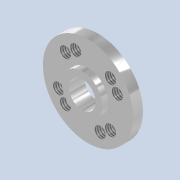
# Autodesk Inventor part: サーボモータ25kgcmサーボホーン1
Saved by Autodesk Inventor 2021.2 (Build 252289000, 289)
## iProperties
Created: 2020-02-02
Part Number: サーボモータ25kgcmサーボホーン1
Material: アルミニウム 6061
Document SubType Name: Modeling
Designer: yuta2
Density: 2.7 g/cm^3
Appearance: アルミニウム - フラット
Mass: 1.75584 g
Surface Area: 8.04248 cm^2
Volume: 0.65031 cm^3
Author: yuta2
Autodesk Inventor part; units mm, degrees
ref_plane "YZ Plane" through (0, 0, 0) normal (1, 0, 0) x (0, 1, 0)
ref_plane "XZ Plane" through (0, 0, 0) normal (0, 1, 0) x (-1, 0, 0)
ref_plane "XY Plane" through (0, 0, 0) normal (0, 0, 1) x (1, 0, 0)
sketch "スケッチ1" plane through (0, 0, 0) normal (0, 0, 1) x (1, 0, 0)
  circle A0 centre (0, 0) radius 10
  dimension "d0" = 20
  constraints: 1 centre point, 1 coincident
  measures "d0" diameter of A0
extrude "押し出し1" add sketch "スケッチ1" along normal blind 2.2
sketch "スケッチ2" plane through (0, 0, 2.2) normal (0, 0, 1) x (1, 0, 0)
  circle A0 centre (0, 0) radius 4.5
  dimension "d3" = 9
  constraints: 1 centre point, 1 coincident
  measures "d3" diameter of A0
extrude "押し出し2" add sketch "スケッチ2" along normal blind 1.3
sketch "スケッチ3" plane through (0, 0, 0) normal (0, 0, -1) x (-1, 0, 0)
  circle A0 centre (0, 0) radius 10 projected
  line L0 (0, 10) -> (0, -10)
  line L1 (-10, 0) -> (10, 0)
  point P0 (-5, 5)
  point P1 (5, 5)
  point P2 (5, -5)
  point P3 (-5, -5)
  dimension "d6" = 10
  dimension "d7" = 10
  constraints: 4 end point, 4 point on circle, 3 midpoint, 3 symmetric about line, 1 perpendicular, 1 vertical
  measures "d6" distance of point (-5, -5) point (-5, 5)
  measures "d7" distance of point (5, 5) point (-5, 5)
hole "穴1" at (5, 5, 0) at (-5, 5, 0) at (-5, -5, 0) at (5, -5, 0) direction (0, 0, 1) diameter 2.459 end through all thread size "M3x0.5" class "6H" standard "ISO Metric profile"
sketch "スケッチ4" plane through (0, 0, 3.5) normal (0, 0, -1) x (-1, 0, 0)
  point P0 (0, 0)
  point P1 (0, 0)
  constraints: 1 coincident
hole "穴2" at (0, 0, 3.5) direction (0, 0, -1) diameter 6 end through all
sketch "スケッチ5" plane through (0, 0, 0) normal (0, 0, -1) x (-1, 0, 0)
  point P0 (-2.7296, -6.523)
  point P1 (2.7296, 6.523)
  point P2 (-6.523, 2.7296)
  point P3 (6.523, -2.7296)
hole "穴3" at (2.7296, -6.523, 0) at (-2.7296, 6.523, 0) at (6.523, 2.7296, 0) at (-6.523, -2.7296, 0) direction (0, 0, 1) diameter 2.459 depth 7 tip angle 120 thread size "M3x0.5" class "6H" standard "ISO Metric profile"
